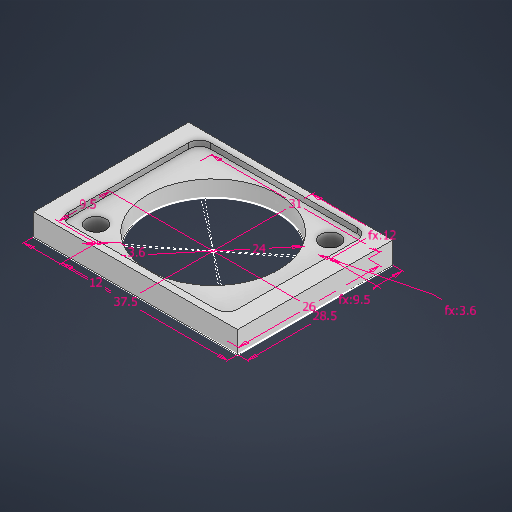
# Autodesk Inventor part: inner clamp plate
Saved by Autodesk Inventor 2026.2 (Build 302298000, 298)
## iProperties
Created: 2026-04-19
Part Number: inner clamp plate
Material: Generic
Document SubType Name: Modeling
Designer: Graeme
Density: 1 g/cm^3
Appearance: Default
Author: Graeme
## iProperties of the stored document inner clamp plate_3DPrint.ipt
Created: 2026-09-26
Part Number: inner clamp plate_3DPrint
Material: Generic
Document SubType Name: Modeling
Designer: Graeme
Density: 1 g/cm^3
Appearance: Default
Author: Graeme
Autodesk Inventor part; units mm, degrees
ref_plane "YZ Plane" through (0, 0, 0) normal (1, 0, 0) x (0, 1, 0)
ref_plane "XZ Plane" through (0, 0, 0) normal (0, 1, 0) x (-1, 0, 0)
ref_plane "XY Plane" through (0, 0, 0) normal (0, 0, 1) x (1, 0, 0)
sketch "Sketch1" plane through (0, 0, 0) normal (0, 1, 0) x (-1, 0, 0)
  line L0 (15.5, 13) -> (-15.5, 13)
  line L1 (-15.5, 13) -> (-15.5, -13)
  line L2 (-15.5, -13) -> (15.5, -13)
  line L3 (15.5, -13) -> (15.5, 13)
  line L4 (15.5, 13) -> (-15.5, -13) construction
  line L5 (-15.5, 13) -> (15.5, -13) construction
  circle A0 centre (0, 0) radius 12
  circle A1 centre (12, 9.5) radius 1.8
  circle A2 centre (-12, -9.5) radius 1.8
  line L6 (18.75, -14.25) -> (-18.75, -14.25)
  line L7 (-18.75, -14.25) -> (-18.75, 14.25)
  line L8 (-18.75, 14.25) -> (18.75, 14.25)
  line L9 (18.75, 14.25) -> (18.75, -14.25)
  line L10 (18.75, -14.25) -> (-18.75, 14.25) construction
  line L11 (-18.75, -14.25) -> (18.75, 14.25) construction
  dimension "d0" = 31
  dimension "d1" = 26
  dimension "d2" = 24
  dimension "d7" = 3.6
  dimension "d8" = 9.5
  dimension "d9" = 12
  dimension "d10" = 3.6
  dimension "d11" = 9.5
  dimension "d12" = 12
  dimension "d16" = 37.5
  dimension "d17" = 28.5
  constraints: 24 end point, 4 midpoint, 4 parallel, 3 centre point, 2 horizontal, 2 perpendicular, 1 coincident
  measures "d0" distance of L2.end L1.end
  measures "d1" distance of L1.end L0.end
  measures "d2" diameter of A0
  measures "d7" diameter of A1
  measures "d8" vertical distance of point (0, 0) A1.centre
  measures "d9" horizontal distance of point (0, 0) A1.centre
  measures "d10" diameter of A2
  measures "d11" vertical distance of point (0, 0) A2.centre
  measures "d12" horizontal distance of A2.centre point (0, 0)
  measures "d16" distance of L7.end L8.end
  measures "d17" distance of L6.end L7.end
extrude "Extrusion2" add sketch "Sketch1" along normal blind 4 contours L3 L2 L1 L0 | L6 L7 L8 L9
sketch "Sketch2" plane through (0, 4, 0) normal (0, 1, 0) x (1, 0, 0)
  line L0 (15.5, 13) -> (-15.5, 13) projected
  line L1 (-15.5, -13) -> (15.5, -13) projected
  line L2 (-18.75, -14.25) -> (18.75, -14.25) projected
  line L3 (18.75, -14.25) -> (18.75, 14.25) projected
  line L4 (18.75, 14.25) -> (-18.75, 14.25) projected
  line L5 (-18.75, 14.25) -> (-18.75, -14.25) projected
  circle A0 centre (0, 0) radius 12 projected
  circle A1 centre (-12, -9.5) radius 1.8 projected
  circle A2 centre (12, 9.5) radius 1.8 projected
  line L6 (15.5, -13) -> (15.5, 13) projected
  line L7 (-15.5, 13) -> (-15.5, -13) projected
extrude "Extrusion3" cut sketch "Sketch2" against normal blind 1 contours L6 L1 L7 L0 | A0 | A1 | A2
fillet "Fillet2" radius 2 4 edges at (-15.5, 3.5, -13) (-15.5, 3.5, 13) (15.5, 3.5, 13) (15.5, 3.5, -13)
equation "\"d10\" = d7"
equation "\"d11\" = d8"
equation "\"d12\" = d9"
body "Solid2"
